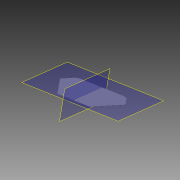
# Autodesk Inventor part: cover
Saved by Autodesk Inventor 2015 SP1 (Build 190203100, 203)
## iProperties
Created: 2015-04-18
Part Number: cover
Material: Ogólny
Document SubType Name: Konstrukcja blachowa
Designer: Marcin
Density: 1 g/cm^3
Sheet Metal Rule: Domyślny
Appearance: Domyślna
Author: Marcin
Autodesk Inventor part; units mm, degrees
ref_plane "YZ Plane" through (0, 0, 0) normal (1, 0, 0) x (0, 1, 0)
ref_plane "XZ Plane" through (0, 0, 0) normal (0, 1, 0) x (-1, 0, 0)
ref_plane "XY Plane" through (0, 0, 0) normal (0, 0, 1) x (1, 0, 0)
ref_plane "Płaszczyzna konstrukcyjna3" through (12.0764, -288.2629, 0.4317) normal (-0.9841767, -0.1771901, 0) x (0.0458602, -0.2547237, -0.9659258)
ref_plane "Płaszczyzna konstrukcyjna9" through (-34.5149, -29.4782, -69.1961) normal (0.0458602, -0.2547237, -0.9659258) x (-0.9841767, -0.1771901, 0)
sketch "Szkic3" plane through (-34.5149, -29.4782, -69.1961) normal (0.0458602, -0.2547237, -0.9659258) x (-0.9841767, -0.1771901, 0)
  line L0 (-83.923, 60) -> (83.923, 60)
  line L1 (83.923, 60) -> (0, 11.547)
  line L2 (0, 11.547) -> (-83.923, 60)
  line L3 (-106.325, 49.8397) -> (-10, -5.7735)
  line L4 (-10, -5.7735) -> (-10, -117)
  line L5 (-10, -117) -> (-67.55, -117)
  line L6 (-67.55, -117) -> (-135.1, 0)
  line L7 (-135.1, 0) -> (-106.325, 49.8397)
  line L8 (152.4205, 0) -> (76.2102, -132)
  line L9 (76.2102, 132) -> (152.4205, 0)
  line L10 (-76.2102, 132) -> (76.2102, 132)
  line L11 (-152.4205, 0) -> (-76.2102, 132)
  line L12 (-76.2102, -132) -> (-152.4205, 0)
  line L13 (76.2102, -132) -> (-76.2102, -132)
  line L14 (10, -117) -> (10, -5.7735)
  line L15 (10, -5.7735) -> (106.325, 49.8397)
  line L16 (106.325, 49.8397) -> (135.1, 0)
  line L17 (135.1, 0) -> (67.55, -117)
  line L18 (67.55, -117) -> (10, -117)
  line L19 (-83.923, 60) -> (-106.325, 49.8397)
  line L20 (-10, -117) -> (10, -117)
  line L21 (106.325, 49.8397) -> (83.923, 60)
  line L22 (83.923, 60) -> (-83.923, 60)
  line L23 (-106.325, 49.8397) -> (-135.1, 0)
  line L24 (-135.1, 0) -> (-67.55, -117)
  line L25 (-67.55, -117) -> (-10, -117)
  line L26 (10, -117) -> (67.55, -117)
  line L27 (67.55, -117) -> (135.1, 0)
  line L28 (135.1, 0) -> (106.325, 49.8397)
  line L29 (84.7877, 64) -> (109.1469, 52.9521)
  line L30 (109.1469, 52.9521) -> (139.7188, 0)
  line L31 (139.7188, 0) -> (69.8594, -121)
  line L32 (69.8594, -121) -> (10, -121)
  line L33 (10, -121) -> (-10, -121)
  line L34 (-10, -121) -> (-69.8594, -121)
  line L35 (-69.8594, -121) -> (-139.7188, 0)
  line L36 (-139.7188, 0) -> (-109.1469, 52.9521)
  line L37 (-109.1469, 52.9521) -> (-84.7877, 64)
  line L38 (-84.7877, 64) -> (84.7877, 64)
  line L39 (83.923, 60) -> (93.6072, 60)
  line L40 (-83.923, 60) -> (-93.6072, 60)
  point P0 (-39.192, 4.2066)
  dimension "d3" = 4
  measures "d3" distance between parallel lines of L21 L29
extrude "Płyta3" add sketch "Szkic3" along normal blind 0.8 contours L0 L1 L2 | L2 L1 L21 L15 L14 L20 L4 L3 L19 | L19 L7 L6 L5 L20 L18 L17 L16 L21 L39 L29 L30 L31 L32 L33 L34 L35 L36 L37 L40 | L3 L4 L5 L6 L7 | L16 L17 L18 L14 L15
sketch "Szkic4" plane through (-34.4782, -29.682, -69.9688) normal (0.0458602, -0.2547237, -0.9659258) x (-0.9841767, -0.1771901, 0)
  circle A0 centre (-12, 40.4) radius 1.5 projected
  circle A1 centre (12, 53.9) radius 1.5 projected
  line L0 (12, 53.9) -> (-12, 53.9) construction
  line L1 (-12, 53.9) -> (-12, 40.4) construction
  line L2 (-12, 40.4) -> (12, 40.4) construction
  line L3 (12, 40.4) -> (12, 53.9) construction
  circle A2 centre (12, 40.4) radius 1.5
  circle A3 centre (-12, 53.9) radius 1.5
  point P0 (-39.192, 4.2066)
  dimension "d5" = 3
  dimension "d6" = 3
  constraints: 8 end point, 2 centre point, 2 coincident, 2 parallel, 1 horizontal, 1 perpendicular
  measures "d5" diameter of A2
  measures "d6" diameter of A3
extrude "Wytnij1" cut sketch "Szkic4" against normal blind 0.8
sketch "Szkic5" plane through (-34.5149, -29.4782, -69.1961) normal (-0.0458602, 0.2547237, 0.9659258) x (0.9841767, 0.1771901, 0)
  point P0 (-12, -108)
  point P1 (12, -108)
hole "Otwór1" at (-27.8405, -134.2738, -41.2436) at (-4.2203, -130.0212, -41.2436) direction (0.0458602, -0.2547237, -0.9659258) diameter 3.4 depth 0.8
equation "\"d7\" = Grubość"
equation "\"PromieńGięcia\" = Grubość"
equation "\"SzerokośćGięciaPodcięcia\" = Grubość"
equation "\"GłębokośćGięciaPodcięcia\" = 0.5 * Grubość"
equation "\"RozmiarPodcięciaNarożnika\" = 4 * Grubość"
equation "\"MinimalnaPozostałość\" = 2 * Grubość"
equation "\"PromieńPrzejścia\" = PromieńGięcia"
equation "\"Rozmiar_promienia_Jacobiego\" = Grubość"
equation "\"Wielk_odstępu\" = Grubość"
equation "\"d0\" = PromieńGięcia"
equation "\"d2\" = PromieńGięcia"
equation "\"d4\" = PromieńGięcia"
equation "\"Grubość\" = 0.8"
